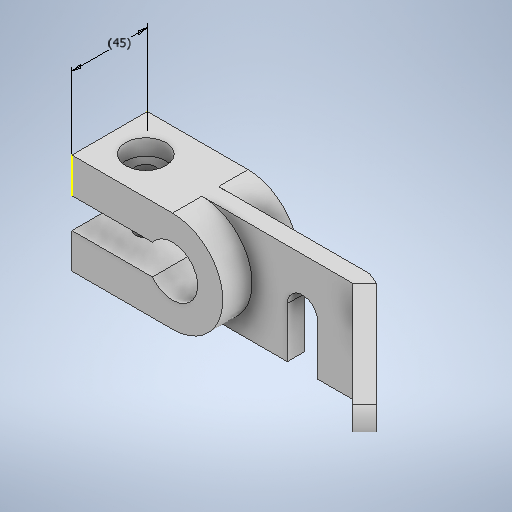
# Autodesk Inventor part: cad@40
Saved by Autodesk Inventor 2025.2 (Build 292293000, 293)
## iProperties
Created: 2025-03-29
Part Number: cad@40
Material: Generic
Document SubType Name: Modeling
Designer: spars
Density: 1 g/cm^3
Appearance: Default
Author: spars
Autodesk Inventor part; units mm, degrees
sketch "Sketch1" plane through (0, 0, 0) normal (0, 0, 1) x (1, 0, 0)
  line L0 (-363.8821, 101.7163) -> (-138.7473, 103.6763) construction
  line L1 (-138.7473, 103.6763) -> (-137.081, -87.7242) construction
  line L2 (-137.081, -87.7242) -> (-362.2158, -89.6841) construction
  line L3 (-362.2158, -89.6841) -> (-363.8821, 101.7163) construction
  line L4 (-45, 30) -> (45, 30)
  line L5 (45, 30) -> (45, -30)
  line L6 (-45, -30) -> (-45, 30)
  line L7 (-45, 30) -> (45, -30) construction
  line L8 (45, 30) -> (-45, -30) construction
  arc A0 (24, 0) -> (6, 0) centre (15, 0) ccw
  line L9 (15, 0) -> (6, 0) construction
  line L10 (15, 0) -> (24, 0) construction
  line L11 (6, 0) -> (6, -30)
  line L12 (24, 0) -> (24, -30)
  line L13 (45, -30) -> (24, -30)
  line L14 (6, -30) -> (-45, -30)
  point P0 (0, 0)
  dimension "d9" = 90
  dimension "d10" = 60
  dimension "d12" = 9
  dimension "d13" = 180
  dimension "d14" = 30
  dimension "d15" = 30
  constraints: 22 end point, 3 parallel, 2 midpoint, 2 point on circle, 1 centre point, 1 horizontal, 1 perpendicular, 2 other
  measures "d9" distance of L5.end L6.start
  measures "d10" distance of L4.end L5.end
  measures "d12" radius of A0
  measures "d13" angle of L9 L10
  measures "d14" distance of L9.end L11.end
  measures "d15" distance of L10.end L12.end
extrude "Extrusion1" add sketch "Sketch1" along normal blind 10
ref_plane "Work Plane1" through (45, -30, 10) normal (0.7071, 0, -0.7071) x (0, 1, 0)
sketch "Sketch2" plane through (45, -30, 10) normal (0.7071, 0, -0.7071) x (0, 1, 0)
  line L0 (60, 0) -> (60, -63.6396) projected
  line L1 (0, 0) -> (60, 0) projected
  circle A0 centre (30, 45.5) radius 7.5
  line L2 (60, 0) -> (36.9322, 55.8626)
  line L3 (0, 0) -> (23.0678, 55.8626)
  arc A1 (36.9322, 55.8626) -> (23.0678, 55.8626) centre (30, 53) ccw
  point P0 (30, -38.8909)
  dimension "d19" = 15
  dimension "d20" = 45.5
  dimension "d22" = 7.5
  constraints: 4 end point, 2 centre point, 2 point on circle, 2 tangent
  measures "d19" diameter of A0
  measures "d20" distance from line of A0.centre L1
  measures "d22" distance of A0.centre A1.centre
extrude "Extrusion2" add sketch "Sketch2" along normal blind 10
sketch "Sketch3" plane through (0, 0, 0) normal (0, 1, 0) x (-1, 0, 0)
  point P0 (0, 0)
sketch "Sketch4" plane through (0, 0, 0) normal (0, 0, 1) x (1, 0, 0)
  point P0 (0, 0)
sketch "Sketch5" plane through (0, 0, 0) normal (0, 1, 0) x (-1, 0, 0)
  point P0 (0, 0)
ref_plane "Work Plane2" through (0, 30, 0) normal (0, 1, 0) x (-1, 0, 0)
ref_plane "Work Plane3" through (0, -30, 0) normal (0, 1, 0) x (-1, 0, 0)
sketch "Sketch6" plane through (0, 30, 0) normal (0, 1, 0) x (-1, 0, 0)
  line L0 (-45, 0) -> (-45, 10) projected
  line L1 (-45, 10) -> (-52.0711, 2.9289) projected
  line L2 (-45, 0) -> (-52.0711, 2.9289)
  line L3 (-52.0711, 2.9289) -> (-45, 10)
  line L4 (-45, 10) -> (-45, 0)
  point P0 (0, 0)
  constraints: 6 end point, 1 collinear, 1 vertical
sketch "Sketch7" plane through (0, -30, 0) normal (0, 1, 0) x (-1, 0, 0)
  point P0 (0, 0)
sketch "Sketch8" plane through (0, -30, 0) normal (0, 1, 0) x (-1, 0, 0)
  line L0 (-45, 10) -> (-52.0711, 2.9289) projected
  line L1 (-52.0711, 2.9289) -> (-45, 10)
  line L2 (-45, 0) -> (-45, 10) projected
  line L3 (-45, 10) -> (-45, 0)
  line L4 (-45, 0) -> (-52.0711, 2.9289)
  point P0 (0, 0)
  constraints: 6 end point, 2 collinear
loft "Loft1" add profiles "Sketch8", "Sketch6"
sketch "Sketch9" plane through (0, 0, 10) normal (0, 0, 1) x (1, 0, 0)
  line L0 (45, 30) -> (-45, 30) projected
  line L1 (-45, 30) -> (-105, 30)
  line L2 (-45, 30) -> (-45, -30) projected
  line L3 (-45, -30) -> (-105, -30)
  arc A0 (-45, -30) -> (-45, 30) centre (-45, 0) ccw
  arc A1 (-57, -9) -> (-57, 9) centre (-45, 0) ccw
  line L4 (-57, 9) -> (-105, 9)
  line L5 (-57, -9) -> (-105, -9)
  line L6 (-105, -30) -> (-105, -9)
  line L7 (-105, 9) -> (-105, 30)
  point P0 (0, 0)
  dimension "d31" = 60
  dimension "d32" = 60
  dimension "d33" = 15
  dimension "d34" = 18
  dimension "d35" = 21
  constraints: 12 end point, 4 horizontal, 4 point on circle, 2 centre point, 1 midpoint
  measures "d31" distance of L0.end L1.end
  measures "d32" distance of L2.end L3.end
  measures "d33" radial gap between concentric circles of A0 A1
  measures "d34" distance between parallel lines of L5 L4
  measures "d35" distance between parallel lines of L3 L5
extrude "Extrusion3" add sketch "Sketch9" along normal blind 17.5 and the other way blind 27.5 contours L2 A1 L4 L7 L1 | A0 L2 A1 | L3 L6 L5 A1 L2
sketch "Sketch10" plane through (-105, 9, 27.5) normal (-1, 0, 0) x (0, 0, 1)
  line L0 (-45, 0) -> (-45, 21) projected
  line L1 (0, 21) -> (0, 0) projected
  point P0 (-27.5, -9)
  point P1 (-45, 10.5)
  dimension "d40" = 45
  constraints: 1 midpoint
  measures "d40" distance from line of point (-45, 10.5) L1
sketch "Sketch11" plane through (-45, 30, 0) normal (0, 1, 0) x (1, 0, 0)
  circle A0 centre (-38.4851, -5) radius 12
  line L0 (0, -27.5) -> (-60, -27.5) projected
  point P0 (45, 0)
  dimension "d42" = 24
  constraints: 1 centre point
  measures "d42" diameter of A0
extrude "Extrusion4" cut sketch "Sketch11" against normal blind 9.5
sketch "Sketch12" plane through (-83.4851, 20.5, 5) normal (0, 1, 0) x (1, 0, 0)
  circle A0 centre (0, 0) radius 12 projected
  circle A1 centre (0, 0) radius 6
  point P0 (83.4851, 5)
  dimension "d46" = 12
  constraints: 1 centre point, 1 coincident
  measures "d46" diameter of A1
extrude "Extrusion5" cut sketch "Sketch12" against normal blind 12 contours A1
sketch "Sketch13" plane through (6, -30, 0) normal (0, -1, 0) x (1, 0, 0)
  circle A0 centre (-89.4851, 5) radius 12
  point P0 (-6, 0)
  dimension "d49" = 24
  constraints: 1 centre point, 1 coincident
  measures "d49" diameter of A0
extrude "Extrusion6" cut sketch "Sketch13" against normal blind 9
sketch "Sketch14" plane through (-83.4851, -21, 5) normal (0, -1, 0) x (1, 0, 0)
  circle A0 centre (0, 0) radius 12 projected
  circle A1 centre (0, 0) radius 6
  point P0 (83.4851, -5)
  dimension "d52" = 12
  constraints: 1 centre point, 1 coincident
  measures "d52" diameter of A1
extrude "Extrusion7" cut sketch "Sketch14" against normal blind 12 contours A1
sketch "Sketch15" plane through (0, 0, 10) normal (0, 0, 1) x (1, 0, 0)
  arc A0 (-45, -15) -> (-45, 15) centre (-45, 0) ccw projected
  line L0 (-45, 15) -> (-45, -15) projected
  line L1 (-45, -15) -> (-45, 15)
  arc A1 (-45, -15) -> (-45, 15) centre (-45, 0) ccw
  point P0 (0, 0)
  constraints: 2 end point, 2 point on circle, 1 centre point, 1 collinear, 1 concentric
extrude "Extrusion8" cut sketch "Sketch15" against normal through all
body "Solid1"
